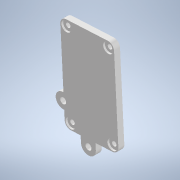
# Autodesk Inventor part: Пластина 2
Saved by Autodesk Inventor 2021 (Build 250183000, 183)
## iProperties
Created: 2020-12-07
Part Number: Пластина 2
Material: Типовые
Document SubType Name: Modeling
Designer: User
Density: 1 g/cm^3
Appearance: По умолчанию
Author: User
Autodesk Inventor part; units mm, degrees
ref_plane "YZ Plane" through (0, 0, 0) normal (1, 0, 0) x (0, 1, 0)
ref_plane "XZ Plane" through (0, 0, 0) normal (0, 1, 0) x (-1, 0, 0)
ref_plane "XY Plane" through (0, 0, 0) normal (0, 0, 1) x (1, 0, 0)
sketch "Эскиз1" plane through (0, 0, 0) normal (0, 0, 1) x (1, 0, 0)
  arc A0 (31.2016, -58.4471) -> (38.772, -50.0394) centre (30.783, -50.4581) ccw projected
  line L0 (31.2016, -58.4471) -> (8.1333, -59.6561) projected
  line L1 (33.0098, 59.9097) -> (38.772, -50.0394) projected
  arc A1 (33.0098, 59.9097) -> (24.6021, 67.4801) centre (25.0208, 59.491) ccw projected
  circle A2 centre (-2.0934, 39.9452) radius 12 projected
  circle A3 centre (0, 0) radius 12 projected
  line L2 (-34.9911, -22.1042) -> (-39.0912, 56.131) projected
  arc A4 (-35.8899, -22.1513) -> (-34.8432, -42.1239) centre (-35.3665, -32.1376) ccw projected
  line L3 (-34.9911, -22.1042) -> (-35.8899, -22.1513) projected
  line L4 (-34.8432, -42.1239) -> (-33.9444, -42.0768) projected
  line L5 (-33.3291, -53.8181) -> (-33.9444, -42.0768) projected
  arc A5 (-33.3291, -53.8181) -> (-24.9213, -61.3884) centre (-25.34, -53.3994) ccw projected
  line L6 (-11.8393, -60.7028) -> (-24.9213, -61.3884) projected
  arc A6 (-31.5209, 64.5388) -> (-39.0912, 56.131) centre (-31.1022, 56.5497) ccw projected
  line L7 (-31.5209, 64.5388) -> (24.6021, 67.4801) projected
  arc A7 (-11.3817, -69.4335) -> (8.5909, -68.3868) centre (-1.3954, -68.9101) ccw projected
  line L8 (-11.8393, -60.7028) -> (-11.3817, -69.4335) projected
  line L9 (8.5909, -68.3868) -> (8.1333, -59.6561) projected
  point P0 (24.6021, 67.4801)
  point P1 (26.2085, -58.7088)
extrude "Выдавливание1" add sketch "Эскиз1" along normal blind 6
sketch "Эскиз2" plane through (0, 0, 6) normal (0, 0, 1) x (1, 0, 0)
  line L0 (38.772, -50.0394) -> (33.0098, 59.9097) projected
  line L1 (8.1333, -59.6561) -> (31.2016, -58.4471) projected
  arc A0 (31.2016, -58.4471) -> (38.772, -50.0394) centre (30.783, -50.4581) ccw projected
  arc A1 (-33.3291, -53.8181) -> (-24.9213, -61.3884) centre (-25.34, -53.3994) ccw projected
  line L2 (-33.9444, -42.0768) -> (-33.3291, -53.8181) projected
  line L3 (-34.8432, -42.1239) -> (-33.9444, -42.0768) projected
  arc A2 (-35.8899, -22.1513) -> (-34.8432, -42.1239) centre (-35.3665, -32.1376) ccw projected
  line L4 (-39.0912, 56.131) -> (-34.9911, -22.1042) projected
  line L5 (-34.9911, -22.1042) -> (-35.8899, -22.1513) projected
  arc A3 (-31.5209, 64.5388) -> (-39.0912, 56.131) centre (-31.1022, 56.5497) ccw projected
  line L6 (24.6021, 67.4801) -> (-31.5209, 64.5388) projected
  arc A4 (33.0098, 59.9097) -> (24.6021, 67.4801) centre (25.0208, 59.491) ccw projected
  arc A5 (-11.3817, -69.4335) -> (8.5909, -68.3868) centre (-1.3954, -68.9101) ccw projected
  line L7 (-11.8393, -60.7028) -> (-11.3817, -69.4335) projected
  line L8 (-24.9213, -61.3884) -> (-11.8393, -60.7028) projected
  line L9 (8.5909, -68.3868) -> (8.1333, -59.6561) projected
  point P0 (0, 0)
extrude "Выдавливание2" add sketch "Эскиз2" along normal blind 2
sketch "Эскиз3" plane through (0, 0, 8) normal (0, 0, 1) x (1, 0, 0)
  circle A0 centre (25.0208, 59.491) radius 3 construction
  circle A1 centre (-31.1022, 56.5497) radius 3 construction
  circle A2 centre (30.783, -50.4581) radius 3 construction
  circle A3 centre (-25.34, -53.3994) radius 3 construction
  point P0 (0, 0)
hole "Отверстие1" at (-25.34, -53.3994, 8) at (30.783, -50.4581, 8) at (-31.1022, 56.5497, 8) at (25.0208, 59.491, 8) direction (0, 0, -1) diameter 6 end through all counterbore diameter 13.5 counterbore depth 2.5 clearance for "болты с шестигранной головкой / гайка ГОСТ 12876-67" size "M6" standard "ГОСТ"
sketch "Эскиз4" plane through (0, 0, 8) normal (0, 0, 1) x (1, 0, 0)
  circle A0 centre (-1.3954, -68.9101) radius 4 construction
  circle A1 centre (-35.3665, -32.1376) radius 4 construction
  point P0 (0, 0)
hole "Отверстие2" at (-1.3954, -68.9101, 8) at (-35.3665, -32.1376, 8) direction (0, 0, -1) diameter 8 end through all clearance for "с потайной головкой ГОСТ 12876-67" size "M8" standard "ГОСТ"
